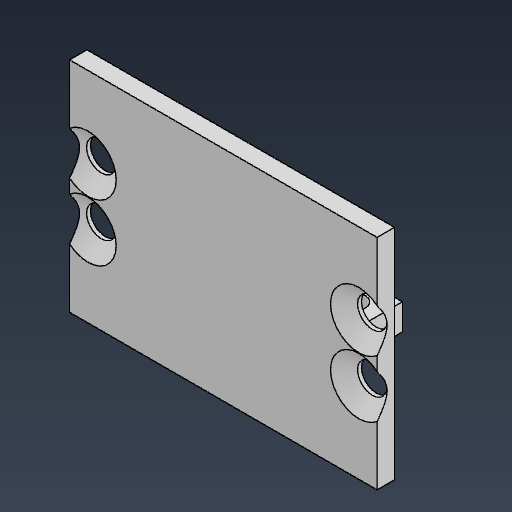
# Autodesk Inventor part: PCB_Holder_Floor
Saved by Autodesk Inventor 2026.2 (Build 302298010, 298A)
## iProperties
Created: 2026-04-05
Part Number: PCB_Holder_Floor
Material: Generic
Document SubType Name: Modeling
Designer: szymo
Density: 1 g/cm^3
Appearance: Default
Author: szymo
Autodesk Inventor part; units mm, degrees
ref_plane "YZ Plane" through (0, 0, 0) normal (1, 0, 0) x (0, 1, 0)
ref_plane "XZ Plane" through (0, 0, 0) normal (0, 1, 0) x (-1, 0, 0)
ref_plane "XY Plane" through (0, 0, 0) normal (0, 0, 1) x (1, 0, 0)
sketch "Sketch1" plane through (0, 0, 0) normal (0, 0, 1) x (1, 0, 0)
  line L0 (-5.85, 27.4958) -> (-32.15, 27.4958) projected
  line L1 (-32.15, 27.4958) -> (-32.15, 26.6958) projected
  line L2 (-32.15, 26.6958) -> (-5.85, 26.6958) projected
  line L3 (-5.85, 26.6958) -> (-5.85, 27.4958) projected
  line L4 (-5.85, 31.2958) -> (-32.15, 31.2958) projected
  line L5 (-32.15, 31.2958) -> (-32.15, 30.4958) projected
  line L6 (-32.15, 30.4958) -> (-5.85, 30.4958) projected
  line L7 (-5.85, 30.4958) -> (-5.85, 31.2958) projected
  line L8 (-1.35, 36.9458) -> (-36.65, 36.9458)
  line L9 (-36.65, 36.9458) -> (-36.65, 23.85)
  line L10 (-36.65, 23.85) -> (-1.35, 23.85)
  line L11 (-1.35, 23.85) -> (-1.35, 36.9458)
  line L12 (-5.95, 27.4958) -> (-11.45, 27.4958)
  line L13 (-11.45, 27.4958) -> (-11.45, 30.4958)
  line L14 (-11.45, 30.4958) -> (-5.95, 30.4958)
  line L15 (-5.95, 30.4958) -> (-5.95, 27.4958)
  line L16 (-26.55, 27.4958) -> (-32.05, 27.4958)
  line L17 (-32.05, 27.4958) -> (-32.05, 30.4958)
  line L18 (-32.05, 30.4958) -> (-26.55, 30.4958)
  line L19 (-26.55, 30.4958) -> (-26.55, 27.4958)
  line L20 (-1.35, 23.85) -> (-1.35, 17.85)
  line L21 (-1.35, 17.85) -> (-36.65, 17.85)
  line L22 (-36.65, 17.85) -> (-36.65, 23.85)
  line L23 (-36.65, 36.9458) -> (-36.65, 42.9458)
  line L24 (-36.65, 42.9458) -> (-1.35, 42.9458)
  line L25 (-1.35, 42.9458) -> (-1.35, 36.9458)
  circle A0 centre (-3.55, 33.6719) radius 2.1 projected
  circle A1 centre (-3.55, 27.124) radius 2.1 projected
  line L26 (-4.75, 23.85) -> (-4.75, 24.5) projected
  line L27 (-1.35, 23.85) -> (-4.75, 23.85) projected
  line L28 (-1.35, 36.9458) -> (-1.35, 23.85) projected
  line L29 (-1.35, 36.9458) -> (-5.15, 36.9458) projected
  line L30 (-5.15, 36.2958) -> (-5.15, 36.9458) projected
  line L31 (-5.15, 36.2958) -> (-5.75, 36.2958) projected
  line L32 (-5.75, 24.5) -> (-5.75, 36.2958) projected
  line L33 (-4.75, 24.5) -> (-5.75, 24.5) projected
  circle A2 centre (-34.45, 27.124) radius 2.1 projected
  circle A3 centre (-34.45, 33.6719) radius 2.1 projected
  line L34 (-33.25, 36.2958) -> (-32.25, 36.2958) projected
  line L35 (-33.25, 36.9458) -> (-33.25, 36.2958) projected
  line L36 (-36.65, 36.9458) -> (-33.25, 36.9458) projected
  line L37 (-36.65, 36.9458) -> (-36.65, 23.85) projected
  line L38 (-36.65, 23.85) -> (-32.25, 23.85) projected
  line L39 (-32.25, 36.2958) -> (-32.25, 23.85) projected
  point P0 (0, 0)
  point P1 (-3.45, 33.6719)
  point P2 (-3.45, 27.124)
  point P3 (-34.55, 27.124)
  point P4 (-34.55, 33.6719)
  point P5 (-26.55, 27.4958)
  point P6 (-11.45, 30.4958)
  point P7 (-11.45, 27.4958)
  point P8 (-31.5, 27.4958)
  point P9 (-7.25, 30.4958)
  dimension "d1" = 5.5
  dimension "d23" = 6
  dimension "d24" = 6
  dimension "d25" = 0
  dimension "d26" = 0
  dimension "d27" = 0
  dimension "d28" = 0
  dimension "d29" = 5.5
  dimension "d30" = 0.2
  dimension "d31" = 0.2
  constraints: 36 end point, 6 parallel, 5 perpendicular, 4 collinear, 4 horizontal, 2 vertical, 1 point on line
  measures "d1" distance between parallel lines of L15 L13
  measures "d23" distance between parallel lines of L21 L10
  measures "d24" distance between parallel lines of L24 L8
  measures "d25" distance between parallel lines of L9 L37
  measures "d26" distance between parallel lines of L11 L28
  measures "d27" distance between parallel lines of L29 L8
  measures "d28" distance between parallel lines of L27 L10
  measures "d29" distance between parallel lines of L19 L17
  measures "d30" distance between parallel lines of L39 L17
  measures "d31" distance between parallel lines of L32 L15
extrude "Extrusion1" add sketch "Sketch1" against normal blind 2 contours L3 L2 L1 L0 | L0 L13 L6 L15 | L0 L19 L6 L13 | L6 L5 L4 L7 | L0 L17 L6 L19 | L11 L10 L26 L33 L32 L31 L30 L8 | L8 L23 L24 L25 | L30 L31 L32 L33 L26 L10 L39 L34 L35 L8 | L20 L21 L22 L10 | L35 L34 L39 L10 L9 L8 | A0 | A1 | A2 | A3
extrude "Extrusion2" add sketch "Sketch1" against normal blind 7.5 contours L0 L13 L6 L15 | L0 L17 L6 L19
sketch "Sketch2" plane through (-11.8, 27.4958, -2) normal (0, -1, 0) x (1, 0, 0)
  line L0 (5.85, -5.5) -> (0.175, 0.175)
  line L1 (0.35, -5.5) -> (5.85, 0)
  line L2 (-14.75, -5.5) -> (-20.25, 0)
  line L3 (-20.25, -5.5) -> (-14.75, 0)
  circle A0 centre (3.1, -2.75) radius 2.75
  circle A1 centre (-17.5, -2.75) radius 2.75
  line L4 (5.85, 0) -> (5.85, -5.5) projected
  line L5 (-20.25, 0) -> (-20.25, -5.5) projected
  line L6 (0.35, -5.5) -> (5.85, -5.5) projected
  line L7 (5.85, -5.5) -> (0.35, -5.5)
  line L8 (-20.25, -5.5) -> (-14.75, -5.5) projected
  line L9 (-20.25, -5.5) -> (-14.75, -5.5)
  point P0 (11.8, 2)
  dimension "d13" = 5.5
  dimension "d14" = 5.5
  constraints: 12 end point, 3 midpoint, 3 point on line, 2 centre point, 2 coincident, 2 collinear, 2 parallel, 1 perpendicular
  measures "d13" diameter of A0
  measures "d14" diameter of A1
hole "Hole1" at (-8.7, 27.4958, -4.75) at (-29.3, 27.4958, -4.75) direction (0, 1, 0) diameter 2.5 end through all
fillet "Fillet1" radius 1 2 edges at (-11.45, 28.9958, -7.5) (-26.55, 28.9958, -7.5)
hole "Hole2" at (-3.45, 27.124, 0) at (-3.45, 33.6719, 0) at (-34.55, 27.124, 0) at (-34.55, 33.6719, 0) direction (0, 0, -1) diameter 3.4 end through all countersink diameter 6.5 countersink angle 90 clearance for "Countersunk Flat Head Screw ISO 2009/7046" size "M3" standard "ISO"
equation "\"d23\" = d24"
equation "\"d29\" = d1"
body "Solid1"
